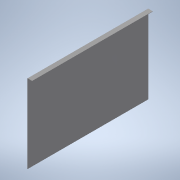
# Autodesk Inventor part: BackWallTop
Saved by Autodesk Inventor 2020 (Build 240168000, 168)
## iProperties
Created: 2025-10-17
Part Number: BackWallTop
Material: Carbon Steel - A36
Document SubType Name: Sheet Metal
Designer: pcajigal
Density: 7.86 g/cm^3
Sheet Metal Rule: 1 HRS Steel
Sheet Metal Width: 0.000 in
Sheet Metal Length: 0.000 in
Sheet Metal Area: 0.000 in^2
Appearance: Steel
Author: pcajigal
Autodesk Inventor part; units mm, degrees
ref_plane "YZ Plane" through (0, 0, 0) normal (1, 0, 0) x (0, 1, 0)
ref_plane "XZ Plane" through (0, 0, 0) normal (0, 1, 0) x (-1, 0, 0)
ref_plane "XY Plane" through (0, 0, 0) normal (0, 0, 1) x (1, 0, 0)
sketch "Sketch29" plane through (0, 0, 0) normal (1, 0, 0) x (0, 1, 0)
  line L0 (0, 0) -> (1657.35, 0)
  line L1 (1657.35, 0) -> (1657.35, 2540)
  line L2 (1657.35, 2540) -> (0, 2540)
  line L3 (0, 2540) -> (0, 0)
  dimension "d230" = 2540
  dimension "d231" = 1657.35
  measures "d230" distance of L0.end L1.end
  measures "d231" distance of L1.end L2.end
extrude "Plate26" add sketch "Sketch29" along normal blind 6.35
sketch "Sketch30" plane through (-0.2216, 1651.0039, 2540) normal (0.0348995, 0.9993908, 0) x (-0.9993908, 0.0348995, 0)
  line L0 (0, -2540) -> (0, 0)
  line L1 (0, 0) -> (-101.6, 0)
  line L2 (-101.6, 0) -> (-101.6, -2540)
  line L3 (-101.6, -2540) -> (0, -2540)
  constraints: 6 end point, 1 horizontal, 1 perpendicular, 1 vertical
edge flange "Flange23" height 101.6 angle 92 thickness 6.35 bend radius 6.35 thickness toward (0.0348995, 0.9993908, 0) relief straight relief width 6.35 relief depth 3.175 edges at (6.35, 1657.35, 1270) wall of the first edge with corners at (-0.2216, 1651.0039, 0) (-0.2216, 1651.0039, 2540) (101.3165, 1647.4581, 2540) (101.3165, 1647.4581, 0)
bend "Bend23"
corner "Corner22"
equation "\"d230\" = LARGO"
equation "\"d231\" = ALTO"
equation "\"d237\" = LARGOF"
equation "\"d238\" = ANGULOF"
equation "\"BendRadius\" = Thickness"
equation "\"BendReliefWidth\" = Thickness"
equation "\"BendReliefDepth\" = 0.5 * Thickness"
equation "\"CornerReliefSize\" = 4 * Thickness"
equation "\"MinimumRemnant\" = 2 * Thickness"
equation "\"TransitionRadius\" = BendRadius"
equation "\"JacobiRadiusSize\" = BendRadius"
equation "\"GapSize\" = Thickness"
equation "\"LARGO\" = 2540"
equation "\"ALTO\" = 1657.35"
equation "\"LARGOF\" = 101.6"
equation "\"ANGULOF\" = 92deg"
body "Solid4"
